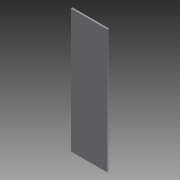
# Autodesk Inventor part: middlehorizotal
Saved by Autodesk Inventor 2011 (Build 150239000, 239)
## iProperties
Created: 2011-11-06
Part Number: middlehorizotal
Document SubType Name: Modeling
Designer: Matthew
Density: 1 g/cm^3
Author: Matthew
Autodesk Inventor part; units mm, degrees
ref_plane "YZ Plane" through (0, 0, 0) normal (1, 0, 0) x (0, 1, 0)
ref_plane "XZ Plane" through (0, 0, 0) normal (0, 1, 0) x (-1, 0, 0)
ref_plane "XY Plane" through (0, 0, 0) normal (0, 0, 1) x (1, 0, 0)
sketch "Sketch1" plane through (0, 0, 0) normal (0, 0, 1) x (1, 0, 0)
  line L0 (-29.7373, 16.182) -> (116.3127, 16.182)
  line L1 (116.3127, 16.182) -> (116.3127, -479.118)
  line L2 (116.3127, -479.118) -> (-29.7373, -479.118)
  line L3 (-29.7373, -479.118) -> (-29.7373, 16.182)
  point P0 (0, 0)
  dimension "d0" = 146.05
  dimension "d1" = 495.3
  constraints: 8 end point, 2 parallel, 1 horizontal, 1 perpendicular
  measures "d0" distance of L1.end L2.end
  measures "d1" distance of L0.end L1.end
extrude "Extrusion1" add sketch "Sketch1" along normal blind 6.35
body "Solid1"
